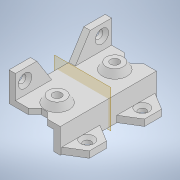
# Autodesk Inventor part: ESC Mount
Saved by Autodesk Inventor 2022 (Build 260153000, 153)
## iProperties
Created: 2022-08-21
Part Number: ESC Mount
Material: Generic
Document SubType Name: Modeling
Designer: Nick
Density: 1 g/cm^3
Appearance: Default
Mass: 4.26085 g
Surface Area: 41.1183 cm^2
Volume: 4.26085 cm^3
Author: Nick
Autodesk Inventor part; units mm, degrees
ref_plane "YZ Plane" through (0, 0, 0) normal (1, 0, 0) x (0, 1, 0)
ref_plane "XZ Plane" through (0, 0, 0) normal (0, 1, 0) x (-1, 0, 0)
ref_plane "XY Plane" through (0, 0, 0) normal (0, 0, 1) x (1, 0, 0)
sketch "Sketch1" plane through (0, 0, 0) normal (0, 0, 1) x (1, 0, 0)
  line L0 (3, 13.65) -> (3, 2.65)
  line L1 (3, 2.65) -> (24, 2.65)
  line L2 (24, 2.65) -> (24, -9)
  line L3 (24, -9) -> (21, -9)
  line L4 (21, -9) -> (21, 0)
  line L5 (21, 0) -> (0, 0)
  line L6 (0, 0) -> (0, 13.65)
  line L7 (0, 13.65) -> (3, 13.65)
  dimension "d0" = 2.65
  dimension "d1" = 21
  dimension "d2" = 9
  dimension "d3" = 3
  dimension "d4" = 3
  dimension "d5" = 11
  constraints: 16 end point, 5 perpendicular, 2 parallel, 1 coincident, 1 vertical
  measures "d0" distance between parallel lines of L5 L1
  measures "d1" distance between parallel lines of L4 L6
  measures "d2" distance between parallel lines of L3 L5
  measures "d3" distance of L2.end L3.end
  measures "d4" distance of L6.end L0.start
  measures "d5" distance of L0.start L0.end
extrude "Extrusion1" add sketch "Sketch1" along normal blind 45
sketch "Sketch2" plane through (3, 2.65, 0) normal (1, 0, 0) x (0, 0, -1)
  line L0 (0, 11) -> (-45, 11) projected
  line L1 (-35, 11) -> (-28, 0)
  line L2 (-17, 0) -> (-10, 11)
  line L3 (0, 0) -> (0, 11) projected
  line L4 (0, 11) -> (-45, 11) projected
  line L5 (-45, 0) -> (-45, 11) projected
  line L6 (0, 0) -> (-45, 0) projected
  point P0 (0, -2.65)
  dimension "d10" = 10
  dimension "d11" = 10
  dimension "d38" = 11
  constraints: 4 end point, 4 point on line, 1 equal length
  measures "d10" distance of L0.end L1.start
  measures "d11" distance of L0.start L2.end
  measures "d38" distance of L2.start L1.end
extrude "Extrusion2" cut sketch "Sketch2" against normal through all contours L2 L6 L1 L0
ref_plane "Work Plane1" through (0, 0, 22.5) normal (0, 0, 1) x (1, 0, 0)
sketch "Sketch3" plane through (3, 2.65, 0) normal (0, 1, 0) x (1, 0, 0)
  line L0 (-3, 0) -> (18, 0) projected
  line L1 (6, 0) -> (9, -3)
  line L2 (9, -3) -> (12, -3)
  line L3 (12, -3) -> (15, 0)
  line L4 (6, -45) -> (9, -42)
  line L5 (9, -42) -> (12, -42)
  line L6 (12, -42) -> (15, -45)
  line L7 (21, 0) -> (0, 0) projected
  line L8 (0, 0) -> (0, -17) projected
  line L9 (0, -17) -> (-3, -17) projected
  line L10 (-3, -28) -> (-3, -17) projected
  line L11 (0, -28) -> (-3, -28) projected
  line L12 (0, -28) -> (0, -45) projected
  line L13 (21, -45) -> (0, -45) projected
  line L14 (21, 0) -> (21, -45) projected
  point P0 (10.5, -3)
  point P1 (10.5, 0)
  point P2 (10.5, -42)
  point P3 (10.5, -45)
  dimension "d14" = 45
  dimension "d15" = 45
  dimension "d16" = 3
  dimension "d17" = 3
  dimension "d18" = 3
  constraints: 12 end point, 4 midpoint, 4 point on line, 3 equal length, 2 horizontal, 2 vertical alignment
  measures "d14" angle of L13 L6
  measures "d15" angle of L7 L3
  measures "d16" distance between parallel lines of L0 L2
  measures "d17" distance between parallel lines of L13 L5
  measures "d18" distance of L4.end L5.end
extrude "Extrusion3" cut sketch "Sketch3" against normal through all contours L0 L3 L2 L1 | L13 L4 L5 L6
sketch "Sketch4" plane through (3, 2.65, 45) normal (1, 0, 0) x (0, 0, -1)
  line L0 (0, 0) -> (0, 11) projected
  line L1 (45, 0) -> (45, 11) projected
  line L2 (45, 11) -> (35, 11) projected
  line L3 (10, 11) -> (0, 11) projected
  point P0 (45, -2.65)
  point P1 (40.5, 5.85)
  point P2 (4.5, 5.85)
  point P3 (0, 5.5)
  point P4 (45, 5.5)
  dimension "d21" = 4.5
  dimension "d22" = 4.5
  dimension "d46" = 5.15
  constraints: 2 midpoint, 1 horizontal alignment
  measures "d21" distance from line of L1 point (40.5, 5.85)
  measures "d22" distance from line of L0 point (4.5, 5.85)
  measures "d46" distance from line of L2 point (40.5, 5.85)
hole "Hole1" at (3, 8.5, 4.5) at (3, 8.5, 40.5) direction (-1, 0, 0) diameter 3.6 end through all countersink diameter 6.3 countersink angle 90 clearance for "Flat Head Machine Screw" size "M3" standard "Ansi Metric M Profile"
sketch "Sketch5" plane through (21, -9, 0) normal (0, -1, 0) x (1, 0, 0)
  line L0 (0, 0) -> (3, 0) projected
  line L1 (3, 0) -> (3, 45) projected
  line L2 (0, 45) -> (3, 45) projected
  line L3 (0, 0) -> (0, 45) projected
  line L4 (3, 0) -> (3, 45) projected
  line L5 (3, 18.5) -> (11, 13.5983)
  line L6 (11, 13.5983) -> (11, 5.5983)
  line L7 (11, 5.5983) -> (3, 0.6965)
  line L8 (3, 44.3035) -> (11, 39.4017)
  line L9 (11, 39.4017) -> (11, 31.4017)
  line L10 (11, 31.4017) -> (3, 26.5)
  point P0 (-21, 0)
  point P1 (3, 22.5)
  point P2 (3, 0.6965)
  dimension "d30" = 8
  dimension "d31" = 8
  dimension "d32" = 8
  dimension "d33" = 8
  dimension "d34" = 4
  dimension "d35" = 4
  constraints: 12 end point, 4 point on line, 2 equal length, 1 midpoint, 1 parallel, 1 vertical
  measures "d30" distance between parallel lines of L1 L9
  measures "d31" distance between parallel lines of L1 L6
  measures "d32" distance of L5.end L6.end
  measures "d33" distance of L8.end L9.end
  measures "d34" distance of L5.start point (3, 22.5)
  measures "d35" distance of L10.end point (3, 22.5)
extrude "Extrusion4" add sketch "Sketch5" against normal blind 3 contours L1 L5 L6 L7 | L8 L9 L10 L1
sketch "Sketch6" plane through (21, -6, 0) normal (0, 1, 0) x (1, 0, 0)
  line L0 (3, -18.5) -> (11, -13.5983) projected
  line L1 (11, -13.5983) -> (11, -5.5983) projected
  line L2 (11, -5.5983) -> (3, -0.6965) projected
  line L3 (3, -18.5) -> (3, -0.6965) projected
  line L4 (3, -44.3035) -> (11, -39.4017) projected
  line L5 (11, -39.4017) -> (11, -31.4017) projected
  line L6 (11, -31.4017) -> (3, -26.5) projected
  line L7 (3, -44.3035) -> (3, -26.5) projected
  point P0 (-21, 0)
  point P1 (6, -35.4017)
  point P2 (6, -9.5983)
  point P3 (7, -16.0491)
  point P4 (7, -28.9509)
  point P5 (11, -35.4017)
  point P6 (11, -9.5983)
  dimension "d62" = 3
  constraints: 4 midpoint, 2 horizontal alignment, 1 vertical alignment
  measures "d62" distance from line of L3 point (6, -9.598)
hole "Hole2" at (27, -6, 35.4017) at (27, -6, 9.5983) direction (0, -1, 0) diameter 3.6 end through all countersink diameter 6.3 countersink angle 90 clearance for "Flat Head Machine Screw" size "M3" standard "Ansi Metric M Profile"
sketch "Sketch7" plane through (24, 2.65, 45) normal (0, 1, 0) x (1, 0, 0)
  circle A0 centre (-10.5, 36) radius 2
  circle A1 centre (-10.5, 9) radius 2
  circle A2 centre (-10.5, 9) radius 4
  circle A3 centre (-10.5, 36) radius 4
  line L0 (-12, 3) -> (-9, 3) projected
  line L1 (-24, 17) -> (-24, 28) projected
  line L2 (-24, 22.5) -> (-9, 22.5) construction
  point P0 (-24, 45)
  point P1 (-10.5, 3)
  dimension "d48" = 4
  dimension "d49" = 13.5
  dimension "d50" = 13.5
  dimension "d51" = 8
  dimension "d61" = 27
  constraints: 4 centre point, 2 coincident, 2 end point, 2 equal radius, 2 midpoint, 2 vertical alignment, 1 horizontal
  measures "d48" diameter of A0
  measures "d49" distance from line of A1.centre L2
  measures "d50" distance from line of A0.centre L2
  measures "d51" diameter of A3
  measures "d61" distance of A0.centre A1.centre
extrude "Extrusion5" add sketch "Sketch7" along normal blind 3
extrude "Extrusion6" cut sketch "Sketch7" against normal through all contours A0 | A1
draft "FaceDraft1" angle 30 pull direction (0, 1, 0) faces at (17.487, 4.65, 36.3219) fixed edges at (9.5, 5.65, 36)
draft "FaceDraft2" angle 30 pull direction (0, 1, 0) faces at (17.487, 4.65, 9.3219) fixed edges at (9.5, 5.65, 9)
equation "\"d21\" = d22"
equation "\"d30\" = d31"
equation "\"d32\" = d31"
equation "\"d33\" = d30"
equation "\"d50\" = d49"
body "Solid1"
